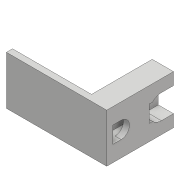
# Autodesk Inventor part: leg_hind_upper_joint
Saved by Autodesk Inventor 2017 (Build 210142000, 142)
## iProperties
Created: 2019-03-28
Part Number: leg_hind_upper_joint
Material: Generic
Document SubType Name: Modeling
Designer: mfans
Density: 1 g/cm^3
Appearance: Default
Author: mfans
Autodesk Inventor part; units mm, degrees
ref_plane "YZ Plane" through (0, 0, 0) normal (1, 0, 0) x (0, 1, 0)
ref_plane "XZ Plane" through (0, 0, 0) normal (0, 1, 0) x (-1, 0, 0)
ref_plane "XY Plane" through (0, 0, 0) normal (0, 0, 1) x (1, 0, 0)
sketch "Sketch1" plane through (0, 0, 0) normal (0, 1, 0) x (-1, 0, 0)
  line L0 (16.5, 8) -> (-16.5, 8)
  line L1 (-16.5, 8) -> (-16.5, -8)
  line L2 (-16.5, -8) -> (16.5, -8)
  line L3 (16.5, -8) -> (16.5, 8)
  line L4 (16.5, 8) -> (-16.5, -8) construction
  line L5 (-16.5, 8) -> (16.5, -8) construction
  point P0 (0, 0)
  dimension "d0" = 16
  dimension "d1" = 33
  constraints: 12 end point, 2 midpoint, 2 parallel, 1 horizontal, 1 perpendicular
  measures "d0" distance between parallel lines of L0 L2
  measures "d1" distance of L1.end L2.end
extrude "Extrusion1" add sketch "Sketch1" along normal blind 2
sketch "Sketch2" plane through (0, 2, 0) normal (0, 1, 0) x (1, 0, 0)
  line L0 (-16.5, -8) -> (16.5, -8) projected
  line L1 (16.5, -8) -> (16.5, 8) projected
  line L2 (16.5, 8) -> (-16.5, 8) projected
  line L3 (-16.5, 8) -> (-16.5, -8) projected
  line L4 (16.5, -8) -> (9.5, -8)
  line L5 (9.5, -8) -> (9.5, 8)
  line L6 (9.5, 8) -> (16.5, 8)
  line L7 (16.5, 8) -> (16.5, -8)
  point P0 (0, 0)
  dimension "d4" = 7
  constraints: 8 end point, 2 parallel, 1 horizontal, 1 perpendicular, 1 point on line
  measures "d4" distance between parallel lines of L1 L5
extrude "Extrusion2" add sketch "Sketch2" along normal blind 20 contours L5 L2 L1 L0
sketch "Sketch3" plane through (16.5, 0, 8) normal (1, 0, 0) x (0, 0, -1)
  line L0 (0, 0) -> (16, 0) projected
  line L1 (16, 0) -> (16, 22) projected
  line L2 (0, 22) -> (16, 22) projected
  line L3 (0, 0) -> (0, 22) projected
  line L4 (10.75, 18) -> (5.25, 18)
  line L5 (5.25, 18) -> (5.25, 2)
  line L6 (5.25, 2) -> (10.75, 2)
  line L7 (10.75, 2) -> (10.75, 18)
  line L8 (10.75, 18) -> (5.25, 2) construction
  line L9 (5.25, 18) -> (10.75, 2) construction
  circle A0 centre (8, 18) radius 4
  line L10 (0, 22) -> (16, 22) projected
  line L11 (4, 18) -> (12, 18)
  line L12 (12, 18) -> (12, 22)
  line L13 (12, 22) -> (4, 22)
  line L14 (4, 22) -> (4, 18)
  point P0 (8, 0)
  point P1 (8, 10)
  dimension "d11" = 8
  dimension "d7" = 4
  dimension "d8" = 16
  dimension "d9" = 5.5
  dimension "d10" = 8
  constraints: 20 end point, 4 parallel, 3 midpoint, 2 horizontal, 2 perpendicular, 1 horizontal alignment, 1 point on line, 2 other
  measures "d7" distance between parallel lines of L2 L4
  measures "d8" distance of L6.end L4.start
  measures "d9" distance between parallel lines of L5 L7
  measures "d10" distance from line of L3 point (8, 10)
extrude "Extrusion3" cut sketch "Sketch3" against normal blind 4 contours A0 L7 L6 L5 | L5 L4 L7 A0
extrude "Extrusion4" cut sketch "Sketch3" against normal blind 5 contours L2 A0 L14 | L12 A0 L2 | A0 L11 L4 | L11 L5 A0 | A0 L7 L11 | L5 L4 L7 A0
sketch "Sketch4" plane through (16.5, 0, 8) normal (1, 0, 0) x (0, 0, -1)
  line L0 (5.25, 2) -> (5.25, 15.0953) projected
  line L1 (10.75, 15.0953) -> (10.75, 2) projected
  line L2 (5.25, 14) -> (10.75, 14)
  line L3 (10.75, 14) -> (10.75, 7.5)
  line L4 (10.75, 7.5) -> (5.25, 7.5)
  line L5 (5.25, 7.5) -> (5.25, 14)
  line L6 (10.75, 2) -> (5.25, 2) projected
  point P0 (8, 0)
  dimension "d16" = 5.5
  dimension "d17" = 6.5
  constraints: 8 end point, 2 parallel, 2 point on line, 1 horizontal, 1 perpendicular
  measures "d16" distance between parallel lines of L4 L6
  measures "d17" distance between parallel lines of L4 L2
extrude "Extrusion5" add sketch "Sketch4" against normal blind 2 contours L0 L2 L1 L4
fillet "Fillet1" radius 2.75 2 edges at (15.5, 7.5, -2.75) (15.5, 7.5, 2.75)
body "Solid1"
